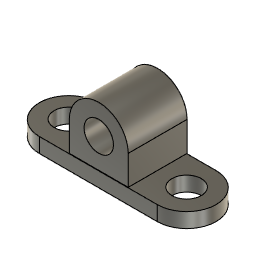
A4 (Autodesk Fusion 360 design; units mm, degrees)
Autodesk Fusion 360 part; units mm, degrees
sketch "Sketch1" plane through (0, 0, 0) normal (0, 0, 1) x (1, 0, 0)
  line L0 (40.3277, 19.712) -> (-39.6723, 19.712)
  line L1 (-39.6723, 19.712) -> (-39.6723, -20.288)
  line L2 (-39.6723, -20.288) -> (40.3277, -20.288)
  line L3 (40.3277, -20.288) -> (40.3277, 19.712)
  line L4 (-39.6723, -0.288) -> (40.3277, -0.288) construction
  circle A0 centre (40, 0) radius 10
  circle A1 centre (-40, 0) radius 10
  line L5 (-24, 12) -> (-20, 10) construction
  line L6 (24, 12) -> (20, 10) construction
  arc A2 (40.3277, -20.288) -> (40.3277, 19.712) centre (40.3277, -0.288) ccw
  arc A3 (-39.6723, 19.712) -> (-39.6723, -20.288) centre (-39.6723, -0.288) ccw
  dimension "d1" = 80
  dimension "d2" = 40
  dimension "d6" = 40
  dimension "d7" = 40
  constraint horizontal L0
  constraint perpendicular L0 L1
  constraint parallel L0 L2
  constraint parallel L1 L3
  constraint coincident origin L6
  constraint coincident origin L5
  constraint midpoint L1 L4.start
  constraint midpoint L3 L4.end
  constraint coincident L4.end A2.centre
  constraint coincident L4.start A3.centre
  measures "d1" distance of L1.end L2.end
  measures "d2" distance of L0.end L1.end
  measures "d6" diameter of A2
  measures "d7" diameter of A3
sketch "Sketch2" plane through (0, 0, 0) normal (0, 0, 1) x (1, 0, 0)
sketch "Sketch3" plane through (0, 0, 0) normal (0, 0, 1) x (1, 0, 0)
extrude "Extrude1" add sketch "Sketch1" along normal blind 10 contours L0 L1 L2 L3 A0 A1 | L3 A0 A2 | L1 A1 A3
sketch "Sketch4" plane through (0, 0, 0) normal (0, 1, 0) x (1, 0, 0)
  line L0 (-19.6723, 0) -> (20.3277, 0)
  line L1 (20.3277, 0) -> (20.3277, -30)
  line L2 (-19.6723, -30) -> (-19.6723, 0)
  line L3 (-39.6723, 0) -> (-39.6723, -10)
  circle A0 centre (0.3277, -30) radius 10
  arc A1 (-19.6723, -30) -> (20.3277, -30) centre (0.3277, -30) ccw
  dimension "d12" = 30
  dimension "d13" = 40
  dimension "d14" = 20
  dimension "d15" = 40
  dimension "d16" = 20
  constraint horizontal L0
  constraint vertical L1
  constraint vertical L2
  constraint concentric A0 A1
  measures "d12" distance of L0.start L2.start
  measures "d13" distance of L1.end L2.start
  measures "d14" distance of L2 L3
  measures "d15" diameter of A1
  measures "d16" diameter of A0
extrude "Extrude2" add sketch "Sketch4" along normal mid plane 40
